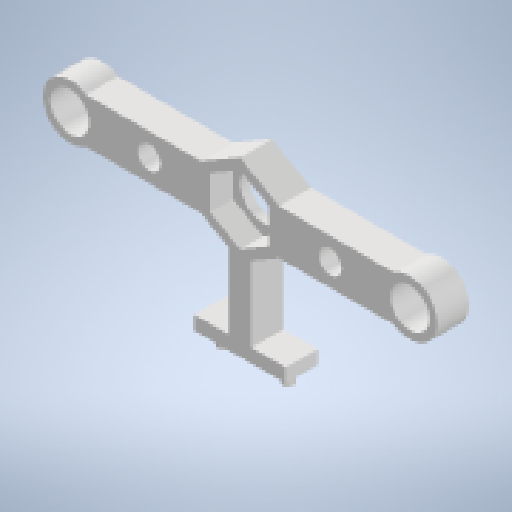
# Autodesk Inventor part: ¸držalo_laserja
Saved by Autodesk Inventor 2023 (Build 270158000, 158)
## iProperties
Created: 2022-09-21
Part Number: ¸držalo_laserja
Material: Generic
Document SubType Name: Modeling
Designer: simon
Density: 1 g/cm^3
Appearance: Default
Author: simon
Autodesk Inventor part; units mm, degrees
ref_plane "YZ Plane" through (0, 0, 0) normal (1, 0, 0) x (0, 1, 0)
ref_plane "XZ Plane" through (0, 0, 0) normal (0, 1, 0) x (-1, 0, 0)
ref_plane "XY Plane" through (0, 0, 0) normal (0, 0, 1) x (1, 0, 0)
sketch "Sketch1" plane through (0, 0, 0) normal (0, 0, 1) x (1, 0, 0)
  circle A0 centre (0, 0) radius 5 projected
  circle A1 centre (0, 0) radius 2.5 projected
  line L0 (33.9967, 2.7031) -> (34.4753, 3.1036) projected
  line L1 (34.4753, 3.1036) -> (34.4758, 3.103) projected
  arc A2 (34.4758, 3.103) -> (34.0516, 2.7031) centre (37, 0) ccw projected
  line L2 (34.0516, 2.7031) -> (33.9967, 2.7031) projected
  circle A3 centre (37, 0) radius 4.25 projected
  circle A4 centre (37, 0) radius 6 projected
  circle A5 centre (-37.0722, -0.0001) radius 4.25 projected
  circle A6 centre (-37, 0) radius 6 projected
  circle A7 centre (0, 0) radius 7.5
  line L3 (0, -7.5) -> (-6.4952, -3.75)
  line L4 (-6.4952, -3.75) -> (-6.4952, 3.75)
  line L5 (-6.4952, 3.75) -> (0, 7.5)
  line L6 (0, 7.5) -> (6.4952, 3.75)
  line L7 (6.4952, 3.75) -> (6.4952, -3.75)
  line L8 (6.4952, -3.75) -> (0, -7.5)
  line L9 (8.4952, -4.9047) -> (8.4952, 4.9047)
  line L10 (8.4952, 4.9047) -> (0, 9.8094)
  line L11 (0, 9.8094) -> (-8.4952, 4.9047)
  line L12 (-8.4952, 4.9047) -> (-8.4952, -4.9047)
  line L13 (-8.4952, -4.9047) -> (0, -9.8094)
  line L14 (0, -9.8094) -> (8.4952, -4.9047)
  line L15 (8.4952, 4.9047) -> (33.544, 4.9047)
  line L16 (8.4952, -4.9047) -> (33.544, -4.9047)
  line L17 (-8.4952, -4.9047) -> (-33.544, -4.9047)
  line L18 (-8.4952, 4.9047) -> (-33.544, 4.9047)
  line L19 (-31, 4.9047) -> (-31, -4.9047)
  line L20 (-31, 4.9047) -> (-8.4952, -4.9047)
  line L21 (31, 0) -> (31, -4.9047)
  line L22 (31, -4.9047) -> (8.4952, 4.9047)
  circle A8 centre (19.7476, 0) radius 2.5
  circle A9 centre (-19.7476, 0) radius 2.5
  line L23 (8.4952, -4.9047) -> (-7.6292, -4.9047)
  line L24 (-0.433, -4.9047) -> (2.067, -4.9047)
  line L25 (2.067, -4.9047) -> (-2.933, -4.9047)
  line L26 (-2.933, -4.9047) -> (-2.933, -24.9047)
  line L27 (-2.933, -24.9047) -> (2.067, -24.9047)
  line L28 (2.067, -24.9047) -> (2.067, -4.9047)
  dimension "d0" = 15
  dimension "d1" = 2
  dimension "d2" = 5
  dimension "d3" = 5
  dimension "d13" = 2.5
  dimension "d14" = 5
  dimension "d15" = 20
  constraints: 52 end point, 7 point on line, 5 point on circle, 4 parallel, 3 horizontal, 3 perpendicular, 2 centre point, 2 coincident, 2 midpoint, 1 tangent, 1 vertical alignment, 20 other
  measures "d1" distance between parallel lines of L7 L9
  measures "d2" diameter of A8
  measures "d3" diameter of A9
  measures "d13" distance of L24.start L24.end
  measures "d14" distance of L27.end L26.end
  measures "d15" distance of L26.end L25.end
extrude "Extrusion1" add sketch "Sketch1" along normal blind 7 contours L23 A7 L3 | L3 L26 A7 L23 | L3 A7 L26 | L23 A7 L28 L8 | L8 A7 L23 | L28 A7 L8 | A7 L26 L13 L12 L11 L10 L9 L23 | A7 L4 | A7 L28 L14 L13 L26 | L7 A7 | L23 L14 L28 A7 | A7 L5 | L6 A7 | L9 L22 A8 L16 | L20 A9 L18 L12 | L17 L19 L20 A9 | L15 A4 L21 L22 A8 | L21 A4 L16 | L17 A6 L19 | A4 | L19 A6 L18 | A6
extrude "Extrusion2" add sketch "Sketch1" along normal blind 2 contours A0 L23 L3 L4 L5 L6 L7 L8 | A0 L23 L28 L8 L3 L26 | L26 L3 L23 | L23 L8 L28
sketch "Sketch4" plane through (0, 0, 7) normal (0, 0, 1) x (1, 0, 0)
  line L0 (-33.544, -4.9047) -> (-8.4952, -4.9047) projected
  line L1 (8.4952, -4.9047) -> (33.544, -4.9047) projected
  arc A0 (33.544, -4.9047) -> (33.544, 4.9047) centre (37, 0) ccw projected
  line L2 (33.544, 4.9047) -> (8.4952, 4.9047) projected
  line L3 (8.4952, 4.9047) -> (0, 9.8094) projected
  line L4 (0, 9.8094) -> (-8.4952, 4.9047) projected
  line L5 (-8.4952, 4.9047) -> (-33.544, 4.9047) projected
  arc A1 (-33.544, 4.9047) -> (-33.544, -4.9047) centre (-37, 0) ccw projected
  circle A2 centre (37, 0) radius 4.25 projected
  circle A3 centre (-19.7476, 0) radius 2.5 projected
  line L6 (6.4952, 3.75) -> (6.4952, -3.75) projected
  line L7 (6.4952, -3.75) -> (0, -7.5) projected
  line L8 (0, -7.5) -> (-6.4952, -3.75) projected
  line L9 (-6.4952, -3.75) -> (-6.4952, 3.75) projected
  line L10 (-6.4952, 3.75) -> (0, 7.5) projected
  line L11 (0, 7.5) -> (6.4952, 3.75) projected
  circle A4 centre (19.7476, 0) radius 2.5 projected
  circle A5 centre (-37.0722, -0.0001) radius 4.25 projected
  line L12 (-8.4952, -4.9047) -> (0, -9.8094) projected
  line L13 (0, -9.8094) -> (8.4952, -4.9047) projected
  line L14 (2.5, 5.1906) -> (-2.5, 5.1906)
  line L15 (-2.5, 5.1906) -> (-2.5, -24.8094)
  line L16 (-2.5, -24.8094) -> (2.5, -24.8094)
  line L17 (2.5, -24.8094) -> (2.5, 5.1906)
  line L18 (2.5, 5.1906) -> (-2.5, -24.8094) construction
  line L19 (-2.5, 5.1906) -> (2.5, -24.8094) construction
  point P0 (0, 0)
  point P1 (2.5, -8.366)
  point P2 (-2.5, -8.366)
  point P3 (0, -24.8094)
  point P4 (0, -24.8094)
  point P5 (2.5, -6.0566)
  point P6 (-2.5, -6.0566)
  dimension "d16" = 5
  dimension "d17" = 30
  constraints: 12 end point, 3 midpoint, 2 parallel, 1 horizontal, 1 perpendicular
  measures "d16" distance of L16.end L15.end
  measures "d17" distance of L15.end L14.end
extrude "Extrusion3" add sketch "Sketch4" against normal blind 7 contours L15 L8 L7 L17 L13 L12 | L12 L13 L17 L16 L15
sketch "Sketch7" plane through (-2.5, -24.8094, 7) normal (0, -1, 0) x (1, 0, 0)
  line L0 (0, 0) -> (5, 0) projected
  line L1 (0, 0) -> (0, -7) projected
  line L2 (5, -7) -> (0, -7) projected
  line L3 (5, 0) -> (5, -7) projected
  line L4 (-7.5, -7) -> (12.5, -7)
  line L5 (12.5, -7) -> (12.5, 0)
  line L6 (12.5, 0) -> (-7.5, 0)
  line L7 (-7.5, 0) -> (-7.5, -7)
  line L8 (2.5, -7) -> (2.5, 0) projected
  line L9 (-7.5, -7) -> (12.5, 0) construction
  line L10 (12.5, -7) -> (-7.5, 0) construction
  point P0 (2.5, -3.5)
  dimension "d24" = 20
  constraints: 12 end point, 3 midpoint, 2 parallel, 2 perpendicular
  measures "d24" distance of L4.start L4.end
extrude "Extrusion5" add sketch "Sketch7" along normal blind 3
sketch "Sketch8" plane through (-2.5, -27.8094, 7) normal (0, -1, 0) x (1, 0, 0)
  line L0 (-7.5, -7) -> (12.5, -7) projected
  line L1 (12.5, -7) -> (12.5, 0) projected
  line L2 (12.5, 0) -> (-7.5, 0) projected
  line L3 (-7.5, 0) -> (-7.5, -7) projected
  line L4 (12.5, -7) -> (12.5, 0) projected
  line L5 (12.5, -3.5) -> (9.5, -3.5)
  circle A0 centre (9.5, -3.5) radius 1.25
  line L6 (-7.5, 0) -> (-7.5, -7) projected
  line L7 (-7.5, -3.5) -> (-4.5, -3.5)
  line L8 (-7.5, -3.5) -> (-4.5, -3.5) construction
  circle A1 centre (-4.5, -3.5) radius 1.25
  point P0 (2.5, -7)
  dimension "d27" = 3
  dimension "d28" = 2.5
  dimension "d29" = 3
  dimension "d30" = 0
  dimension "d31" = 2.5
  constraints: 6 end point, 3 horizontal, 2 centre point, 2 coincident, 2 midpoint, 1 collinear
  measures "d27" distance of L5.start L5.end
  measures "d28" diameter of A0
  measures "d29" distance of L7.start L7.end
  measures "d30" distance between parallel lines of L7 L8
  measures "d31" diameter of A1
extrude "Extrusion6" add sketch "Sketch8" along normal blind 3 contours A0 | A1
body "Solid1"
